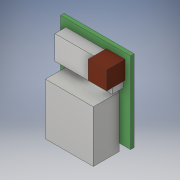
# Autodesk Inventor part: Battery-Management
Saved by Autodesk Inventor 2019 (Build 230136000, 136)
## iProperties
Created: 2018-11-25
Part Number: Battery-Management
Material: Generic
Document SubType Name: Modeling
Designer: lateSWE
Density: 1 g/cm^3
Appearance: Default
Author: lateSWE
Autodesk Inventor part; units mm, degrees
ref_plane "YZ Plane" through (0, 0, 0) normal (1, 0, 0) x (0, 1, 0)
ref_plane "XZ Plane" through (0, 0, 0) normal (0, 1, 0) x (-1, 0, 0)
ref_plane "XY Plane" through (0, 0, 0) normal (0, 0, 1) x (1, 0, 0)
sketch "Sketch1" plane through (0, 0, 0) normal (0, 0, 1) x (1, 0, 0)
  line L0 (0, 0) -> (19, 0)
  line L1 (19, 0) -> (19, 22)
  line L2 (19, 22) -> (0, 22)
  line L3 (0, 22) -> (0, 0)
  dimension "d0" = 19
  dimension "d1" = 22
  constraints: 8 end point, 2 parallel, 1 horizontal, 1 perpendicular
  measures "d0" distance of L2.end L1.end
  measures "d1" distance of L1.end L0.end
extrude "Extrusion1" add sketch "Sketch1" along normal blind 1
sketch "Sketch2" plane through (0, 0, 1) normal (0, 0, 1) x (1, 0, 0)
  line L0 (0, 0) -> (19, 0) projected
  line L1 (0, 0) -> (2.9, 0)
  line L2 (2.9, 0) -> (2.9, 12)
  line L3 (2.9, 12) -> (0, 12)
  line L4 (0, 12) -> (0, 0)
  line L5 (2.9, 12) -> (15.9, 12)
  line L6 (15.9, 12) -> (15.9, -2)
  line L7 (15.9, -2) -> (2.9, -2)
  line L8 (2.9, -2) -> (2.9, 12)
  dimension "d4" = 2.9
  dimension "d5" = 12
  dimension "d6" = 13
  dimension "d7" = 14
  constraints: 16 end point, 4 parallel, 2 horizontal, 2 perpendicular
  measures "d4" distance of L3.end L2.end
  measures "d5" distance of L2.end L1.end
  measures "d6" distance of L6.end L7.end
  measures "d7" distance of L5.end L6.end
extrude "Extrusion2" add sketch "Sketch2" along normal blind 7 contours L2 L5 L6 L0 | L0 L6 L7 L8
sketch "Sketch3" plane through (0, 0, 0) normal (0, 0, -1) x (-1, 0, 0)
  line L0 (-19, 0) -> (-19, 22) projected
  line L1 (-19, 0) -> (-13.5, 0)
  line L2 (-13.5, 0) -> (-13.5, 5)
  line L3 (-13.5, 5) -> (-19, 5)
  line L4 (-19, 5) -> (-19, 0)
  line L5 (-13.5, 0) -> (-5.5, 0)
  line L6 (-5.5, 0) -> (-5.5, 5.5)
  line L7 (-5.5, 5.5) -> (-13.5, 5.5)
  line L8 (-13.5, 5.5) -> (-13.5, 0)
  line L9 (-13.5, 0) -> (-5.5, 0)
  line L10 (-5.5, 0) -> (-5.5, -1.5)
  line L11 (-5.5, -1.5) -> (-13.5, -1.5)
  line L12 (-13.5, -1.5) -> (-13.5, 0)
  point P0 (0, 0)
  dimension "d10" = 5.5
  dimension "d11" = 5
  dimension "d12" = 8
  dimension "d13" = 5.5
  dimension "d16" = 8
  dimension "d17" = 1.5
  constraints: 24 end point, 6 parallel, 3 horizontal, 3 perpendicular
  measures "d10" distance of L3.end L2.end
  measures "d11" distance of L2.end L1.end
  measures "d12" distance of L7.end L6.end
  measures "d13" distance of L6.end L5.end
  measures "d16" distance of L10.end L11.end
  measures "d17" distance of L9.end L10.end
extrude "Extrusion3" add sketch "Sketch3" along normal blind 3 contours L2 L8 L7 L6 L5 | L5 L10 L11 L12
sketch "Sketch4" plane through (0, 0, 1) normal (0, 0, 1) x (1, 0, 0)
  line L0 (19, 22) -> (0, 22) projected
  line L1 (0, 22) -> (1.5, 22)
  line L2 (1.5, 22) -> (1.5, 20.5)
  line L3 (1.5, 20.5) -> (0, 20.5)
  line L4 (0, 20.5) -> (0, 22)
  line L5 (19, 22) -> (17.5, 22)
  line L6 (17.5, 22) -> (17.5, 20.5)
  line L7 (17.5, 20.5) -> (19, 20.5)
  line L8 (19, 20.5) -> (19, 22)
  line L9 (17.5, 20.5) -> (1.5, 20.5)
  line L10 (1.5, 20.5) -> (1.5, 13.5)
  line L11 (1.5, 13.5) -> (17.5, 13.5)
  line L12 (17.5, 13.5) -> (17.5, 20.5)
  point P0 (0, 0)
  dimension "d18" = 1.5
  dimension "d19" = 1.5
  dimension "d20" = 1.5
  dimension "d21" = 1.5
  dimension "d22" = 16
  dimension "d23" = 7
  constraints: 24 end point, 6 parallel, 3 horizontal, 3 perpendicular
  measures "d18" distance of L2.end L3.end
  measures "d19" distance of L1.end L2.end
  measures "d20" distance of L7.end L6.end
  measures "d21" distance of L6.end L5.end
  measures "d22" distance of L11.end L10.end
  measures "d23" distance of L10.end L9.end
extrude "Extrusion4" add sketch "Sketch4" along normal blind 3 contours L12 L11 L10 L9
sketch "Sketch5" plane through (0, 0, 4) normal (0, 0, 1) x (1, 0, 0)
  line L0 (17.5, 20.5) -> (1.5, 20.5) projected
  line L1 (17.5, 20.5) -> (12.5, 20.5)
  line L2 (12.5, 20.5) -> (12.5, 15.5)
  line L3 (12.5, 15.5) -> (17.5, 15.5)
  line L4 (17.5, 15.5) -> (17.5, 20.5)
  point P0 (0, 0)
  dimension "d26" = 5
  dimension "d27" = 5
  constraints: 8 end point, 2 parallel, 1 horizontal, 1 perpendicular
  measures "d26" distance of L3.end L2.end
  measures "d27" distance of L2.end L1.end
extrude "Extrusion5" add sketch "Sketch5" along normal blind 2
sketch "Sketch6" plane through (1.5, 20.5, 1) normal (0, 1, 0) x (1, 0, 0)
  line L0 (0, -3) -> (16, -3) projected
  line L1 (0, -3) -> (11, -3)
  line L2 (11, -3) -> (11, 0)
  line L3 (11, 0) -> (0, 0)
  line L4 (0, 0) -> (0, -3)
  point P0 (-1.5, 1)
  dimension "d30" = 11
  dimension "d31" = 3
  constraints: 8 end point, 2 parallel, 1 horizontal, 1 perpendicular
  measures "d30" distance of L3.end L2.end
  measures "d31" distance of L2.end L1.end
extrude "Extrusion6" cut sketch "Sketch6" against normal blind 0.5
sketch "Sketch7" plane through (17.5, 13.5, 1) normal (1, 0, 0) x (0, 0, -1)
  line L0 (0, 0) -> (-3, 0) projected
  line L1 (-3, 0) -> (0, 0)
  line L2 (0, 0) -> (0, 2)
  line L3 (0, 2) -> (-3, 2)
  line L4 (-3, 2) -> (-3, 0)
  point P0 (1, -13.5)
  dimension "d34" = 3
  dimension "d35" = 2
  constraints: 8 end point, 2 parallel, 1 horizontal, 1 perpendicular
  measures "d34" distance of L3.end L2.end
  measures "d35" distance of L2.end L1.end
extrude "Extrusion7" cut sketch "Sketch7" against normal blind 0.5
body "Solid1"
